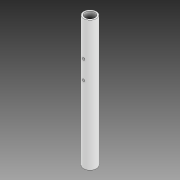
# Autodesk Inventor part: FE-110-005 Inside Connector Bar
Saved by Autodesk Inventor 2021 (Build 250183000, 183)
## iProperties
Created: 2021-01-11
Part Number: FE-110-005 Inside Connector Bar
Material: PVC-Piping
Document SubType Name: Modeling
Density: 1.4 g/cm^3
Appearance: Smooth - White
Autodesk Inventor part; units mm, degrees
ref_plane "YZ Plane" through (0, 0, 0) normal (1, 0, 0) x (0, 1, 0)
ref_plane "XZ Plane" through (0, 0, 0) normal (0, 1, 0) x (-1, 0, 0)
ref_plane "XY Plane" through (0, 0, 0) normal (0, 0, 1) x (1, 0, 0)
sketch "Sketch1" plane through (0, 0, 0) normal (0, 1, 0) x (-1, 0, 0)
  circle A0 centre (0, 0) radius 13.335
  circle A1 centre (0, 0) radius 17.526
  dimension "d0" = 26.67
  dimension "d1" = 35.052
  constraints: 2 centre point, 2 coincident
  measures "d0" diameter of A0
  measures "d1" diameter of A1
extrude "Extrusion1" add sketch "Sketch1" along normal mid plane 355.6
sketch "Sketch3" plane through (0, 0, 0) normal (0, 0, 1) x (1, 0, 0)
  circle A0 centre (0, 31.75) radius 3.175
  circle A1 centre (0, 82.55) radius 3.175
  line L0 (-13.335, 177.8) -> (13.335, 177.8) projected
  point P0 (0, 0)
  dimension "d12" = 6.35
  dimension "d15" = 50.8
  dimension "d16" = 95.25
  constraints: 2 centre point, 2 vertical alignment, 1 equal radius
  measures "d12" diameter of A0
  measures "d15" distance of A0.centre A1.centre
  measures "d16" distance from line of L0 A1.centre
extrude "Extrusion3" cut sketch "Sketch3" against normal through all both and the other way through all
body "Solid1"
